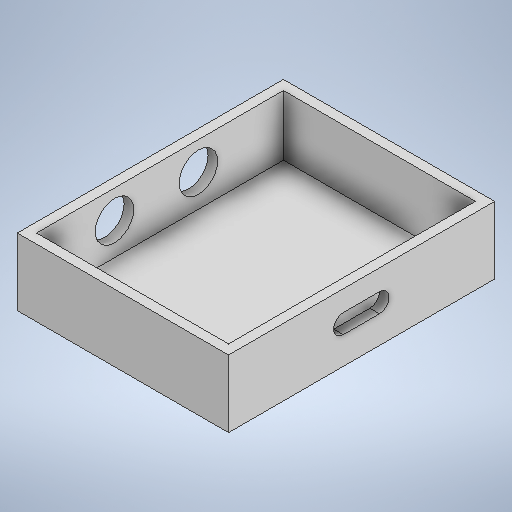
# Autodesk Inventor part: Part2
Saved by Autodesk Inventor 2025.1 (Build 291241000, 241)
## iProperties
Created: 2026-04-18
Part Number: Part2
Material: Generic
Document SubType Name: Modeling
Designer: Luke Buonanno
Density: 1 g/cm^3
Appearance: Default
Author: Luke Buonanno
Autodesk Inventor part; units mm, degrees
ref_plane "YZ Plane" through (0, 0, 0) normal (1, 0, 0) x (0, 1, 0)
ref_plane "XZ Plane" through (0, 0, 0) normal (0, 1, 0) x (-1, 0, 0)
ref_plane "XY Plane" through (0, 0, 0) normal (0, 0, 1) x (1, 0, 0)
sketch "Sketch1" plane through (0, 0, 0) normal (0, 1, 0) x (-1, 0, 0)
  line L0 (-19.25, 24.25) -> (19.25, 24.25)
  line L1 (19.25, 24.25) -> (19.25, -24.25)
  line L2 (19.25, -24.25) -> (-19.25, -24.25)
  line L3 (-19.25, -24.25) -> (-19.25, 24.25)
  line L4 (-19.25, 24.25) -> (19.25, -24.25) construction
  line L5 (19.25, 24.25) -> (-19.25, -24.25) construction
  point P0 (0, 0)
  dimension "d0" = 38.5
  dimension "d1" = 48.5
  constraints: 12 end point, 2 midpoint, 2 parallel, 1 horizontal, 1 perpendicular
  measures "d0" distance of L1.end L2.end
  measures "d1" distance of L2.end L0.start
extrude "Extrusion1" add sketch "Sketch1" along normal blind 12.25
sketch "Sketch2" plane through (0, 12.25, 0) normal (0, 1, 0) x (1, 0, 0)
  line L0 (-17.5, -22.5) -> (17.5, -22.5)
  line L1 (17.5, -22.5) -> (17.5, 22.5)
  line L2 (17.5, 22.5) -> (-17.5, 22.5)
  line L3 (-17.5, 22.5) -> (-17.5, -22.5)
  line L4 (-17.5, -22.5) -> (17.5, 22.5) construction
  line L5 (17.5, -22.5) -> (-17.5, 22.5) construction
  point P0 (0, 0)
  dimension "d4" = 35
  dimension "d5" = 45
  constraints: 12 end point, 2 midpoint, 2 parallel, 1 horizontal, 1 perpendicular
  measures "d4" distance of L1.end L2.end
  measures "d5" distance of L0.end L1.end
extrude "Extrusion2" cut sketch "Sketch2" against normal blind 11
sketch "Sketch3" plane through (19.25, 0, 24.25) normal (1, 0, 0) x (0, 0, -1)
  line L0 (46.75, 1.25) -> (1.75, 1.25) projected
  line L1 (46.75, 12.25) -> (46.75, 1.25) projected
  line L2 (1.75, 12.25) -> (1.75, 1.25) projected
  line L3 (1.75, 8.5) -> (19.15, 8.5)
  line L4 (46.75, 8.5) -> (29.25, 8.5)
  line L5 (19.15, 1.25) -> (19.15, 5)
  line L6 (19.15, 5) -> (29.25, 5)
  line L7 (29.25, 5) -> (29.25, 8.5)
  line L8 (29.25, 8.5) -> (19.15, 8.5)
  line L9 (19.15, 8.5) -> (19.15, 5)
  circle A0 centre (20.9, 6.75) radius 1.75
  circle A1 centre (27.5, 6.75) radius 1.75
  point P0 (24.25, 0)
  point P1 (20.9, 5)
  point P2 (27.5, 5)
  point P3 (27.5, 8.5)
  point P4 (20.9, 8.5)
  dimension "d8" = 17.4
  dimension "d9" = 17.5
  dimension "d10" = 3.75
  dimension "d11" = 3.75
  dimension "d12" = 3.75
  dimension "d22" = 0
  constraints: 14 end point, 6 tangent, 3 horizontal, 3 point on line, 2 centre point, 2 parallel, 1 perpendicular, 1 vertical
  measures "d8" distance of L3.start L3.end
  measures "d9" distance of L4.start L4.end
  measures "d10" distance of L5.start L5.end
  measures "d11" distance of L2.start L3.start
  measures "d12" distance of L1.start L4.start
  measures "d22" distance of L8.end L3.end
extrude "Extrusion3" cut sketch "Sketch3" against normal blind 11 contours A0 L8 A1 L6 | A0 | A1
sketch "Sketch4" plane through (-19.25, 0, -24.25) normal (-1, 0, 0) x (0, 0, 1)
  line L0 (46.75, 1.25) -> (1.75, 1.25) projected
  line L1 (1.75, 12.25) -> (1.75, 1.25) projected
  line L2 (46.75, 12.25) -> (46.75, 1.25) projected
  line L3 (24.25, 1.25) -> (24.25, 6.36)
  line L4 (1.75, 7.11) -> (17.25, 7.11)
  line L5 (46.75, 7.11) -> (32.55, 7.11)
  circle A0 centre (17.25, 7.11) radius 3.504
  circle A1 centre (32.55, 7.11) radius 3.504
  point P0 (24.25, 0)
  dimension "d23" = 5.11
  dimension "d24" = 15.5
  dimension "d25" = 14.2
  constraints: 6 end point, 2 centre point, 2 coincident, 2 point on line, 1 horizontal, 1 midpoint, 1 perpendicular, 1 vertical
  measures "d23" distance of L3.start L3.end
  measures "d24" distance of L4.start L4.end
  measures "d25" distance of L5.start L5.end
extrude "Extrusion4" cut sketch "Sketch4" against normal blind 11
body "Solid1"
